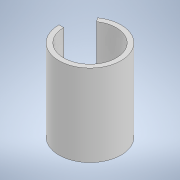
# Autodesk Inventor part: flute-wrapper
Saved by Autodesk Inventor 2022 (Build 260153000, 153)
## iProperties
Created: 2021-09-28
Part Number: flute-wrapper
Material: Generic
Document SubType Name: Modeling
Designer: royja
Density: 1 g/cm^3
Appearance: Default
Author: royja
Autodesk Inventor part; units mm, degrees
ref_plane "YZ Plane" through (0, 0, 0) normal (1, 0, 0) x (0, 1, 0)
ref_plane "XZ Plane" through (0, 0, 0) normal (0, 1, 0) x (-1, 0, 0)
ref_plane "XY Plane" through (0, 0, 0) normal (0, 0, 1) x (1, 0, 0)
sketch "Sketch1" plane through (0, 0, 0) normal (0, 1, 0) x (-1, 0, 0)
  circle A0 centre (0, 0) radius 12.9
  dimension "d0" = 25.8
  constraints: 1 centre point, 1 coincident
  measures "d0" diameter of A0
extrude "Extrusion1" add sketch "Sketch1" along normal blind 34
sketch "Sketch2" plane through (0, 34, 0) normal (0, 1, 0) x (1, 0, 0)
  circle A0 centre (0, 0) radius 10.925
  dimension "d3" = 21.85
  constraints: 1 centre point, 1 coincident
  measures "d3" diameter of A0
extrude "Extrusion2" cut sketch "Sketch2" against normal through all
sketch "Sketch3" plane through (0, 34, 0) normal (0, 1, 0) x (1, 0, 0)
  circle A0 centre (0, 0) radius 12.9 projected
  arc A1 (-7.3991, 10.5671) -> (-12.9, 0) centre (0, 0) ccw
  line L0 (0, 0) -> (-7.3991, 10.5671) construction
  line L1 (0, 0) -> (-12.9, 0) construction
  line L2 (-12.9, 0) -> (0, 0)
  line L3 (0, 0) -> (-7.3991, 10.5671)
  dimension "d6" = 55
  constraints: 8 end point, 3 point on circle, 2 collinear, 1 centre point, 1 coincident
  measures "d6" angle of L0 L1
extrude "Extrusion3" cut sketch "Sketch3" against normal through all contours L3 L2 A0 picked at (-5.6993, 6.3576)
body "Solid1"
